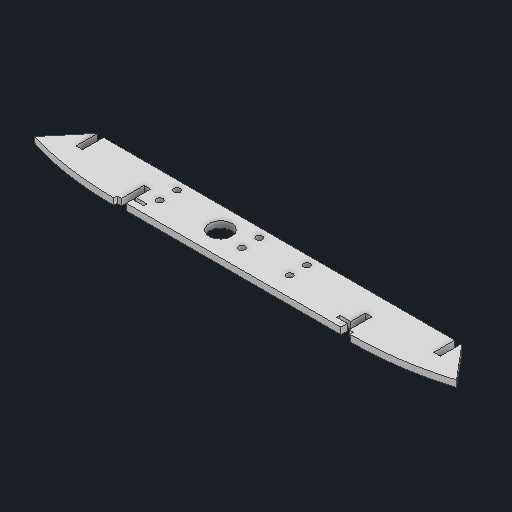
# Autodesk Inventor part: transom
Saved by Autodesk Inventor 2024 (Build 280153000, 153)
## iProperties
Created: 2022-03-21
Part Number: transom
Material: Generic
Document SubType Name: Modeling
Designer: kardo
Density: 1 g/cm^3
Appearance: Default
Mass: 10.6651 g
Surface Area: 88.9068 cm^2
Volume: 10.6651 cm^3
Author: kardo
Autodesk Inventor part; units mm, degrees
ref_plane "YZ Plane" through (0, 0, 0) normal (1, 0, 0) x (0, 1, 0)
ref_plane "XZ Plane" through (0, 0, 0) normal (0, 1, 0) x (-1, 0, 0)
ref_plane "XY Plane" through (0, 0, 0) normal (0, 0, 1) x (1, 0, 0)
derived "parameters_frame.ipt"
derived "stencil_frame.ipt"
sketch "sk_joint_locations" plane through (81.12, 0, 0) normal (1, 0, 0) x (0, 1, 0)
  line L0 (0, 0) -> (122.4, 9.6331) construction
  line L1 (36.465, 28.832) -> (112.2, 28.832) construction
  arc A0 (36.465, 28.832) -> (11.22, 28.376) centre (36.465, -670.197) ccw construction
  line L2 (-241.5001, 19.2432) -> (11.22, 28.376) construction
  line L3 (-345, 16.32) -> (-262.2001, 18.586) construction
  arc A1 (-262.2001, 18.586) -> (-241.5001, 19.2432) centre (-326.8578, 2381.2399) ccw construction
  line L4 (-122.4795, 3121.122) -> (270.8781, -1876.9598) construction
  line L5 (-230.0001, 3089.1136) -> (-230.0001, -1866.0023) construction
  line L6 (-114.9999, 3089.1136) -> (-114.9999, -1866.0023) construction
  line L7 (-345, 3089.1136) -> (-345, -1866.0023) construction
  line L8 (0, 3089.1136) -> (0, -1866.0023) construction
  line L9 (529.622, 47.2379) -> (-602.608, 2.7525) construction
  line L10 (-673.1615, -36.5999) -> (647.9226, 67.3717) construction
  line L11 (189.4528, 29.5173) -> (189.1111, 38.2146) construction
  line L12 (201.105, 36.5853) -> (201.7901, 27.8813) construction
  line L13 (0, 14.144) -> (121.9006, 15.9783) construction
  line L14 (-230.0001, 45.8224) -> (-230.0001, 19.6588) construction
  line L15 (-345, 37.3935) -> (-345, 16.32) construction
  line L16 (-114.9999, 50.9907) -> (-114.9999, 23.8147) construction
  line L17 (0, 52.89) -> (0, 27.9705) construction
  line L18 (119.1768, 50.5875) -> (119.7216, 43.6656) construction
  line L19 (120.2663, 36.7438) -> (119.7216, 43.6656) construction
  line L20 (120.2663, 36.7438) -> (120.8111, 29.822) construction
  line L21 (120.8111, 29.822) -> (121.3559, 22.9001) construction
  line L22 (121.3559, 22.9001) -> (121.9006, 15.9783) construction
  line L23 (0, 14.144) -> (0, 0) construction
  spline S0 degree 4 poles (-345, 37.3935) (-258.8686, 45.1235) (-172.5923, 49.7074) (-86.3167, 52.89) (0, 52.89) knots 0 0 0 0 0 1 1 1 1 1
  spline S1 degree 3 poles (0, 52.89) (92.8353, 52.89) (195.0311, 49.5089) (255, 36.448) knots 0 0 0 0 1 1 1 1
  spline S2 degree 2 poles (122.4, 9.6331) (190.08, 14.9596) (255, 36.448) knots 0 0 0 1 1 1
  line L24 (112.2, 37.536) -> (112.2, 28.832) construction
  line L25 (112.2, 35.848) -> (112.2, 30.52) construction
  point P0 (-122.4795, 3121.122)
  point P1 (270.8781, -1876.9598)
  point P2 (189.282, 33.8659)
  point P3 (201.4475, 32.2333)
  point P4 (134.9575, 11.3411)
  point P5 (-345, 26.8568)
  point P6 (-230.0001, 32.7406)
  point P7 (-114.9999, 37.4027)
  point P8 (0, 40.4303)
  point P9 (112.2, 33.184)
sketch "sk_rudder_mount" plane through (0, -345, 0) normal (0, 1, 0) x (-1, 0, 0)
  line L0 (54.6, -1866.0023) -> (54.6, 3089.1136) construction
  line L1 (0, 16.32) -> (54.6, 16.32) construction
  line L2 (43, 29.32) -> (43, 21.32) construction
  point P0 (0, 0)
  point P1 (0, 39.712)
sketch3d "sk_servo_rod"
sketch "sk_cowl_joint_locations" plane through (54.6, 0, 0) normal (1, 0, 0) x (0, 1, 0)
  line L0 (-345, 16.32) -> (-262.2001, 18.586) construction
  arc A0 (-262.2001, 18.586) -> (-241.5001, 19.2432) centre (-326.8578, 2381.2399) ccw construction
  line L1 (-241.5001, 19.2432) -> (11.22, 28.376) construction
  arc A1 (36.465, 28.832) -> (11.22, 28.376) centre (36.465, -670.197) ccw construction
  line L2 (36.465, 28.832) -> (112.2, 28.832) construction
  line L3 (94.8, 29.632) -> (36.465, 29.632) construction
  arc A2 (36.465, 29.632) -> (11.1911, 29.1755) centre (36.465, -670.197) ccw construction
  line L4 (11.1911, 29.1755) -> (-241.529, 20.0427) construction
  arc A3 (-262.222, 19.3857) -> (-241.529, 20.0427) centre (-326.8578, 2381.2399) ccw construction
  line L5 (-262.222, 19.3857) -> (-345, 17.1203) construction
  line L6 (-230.0001, 3089.1136) -> (-230.0001, -1866.0023) construction
  line L7 (-114.9999, 3089.1136) -> (-114.9999, -1866.0023) construction
  line L8 (-345, 3089.1136) -> (-345, -1866.0023) construction
  line L9 (0, 3089.1136) -> (0, -1866.0023) construction
  line L10 (-230.0001, 44.8681) -> (-230.0001, 20.4593) construction
  line L11 (-114.9999, 49.7658) -> (-114.9999, 24.6152) construction
  line L12 (-345, 17.1203) -> (-345, 17.1203)
  line L13 (-345, 17.1203) -> (-345, 36.7228) construction
  line L14 (-850.7464, 3011.9134) -> (325.2296, -1886.3794) construction
  line L15 (-344.7454, 36.7228) -> (-345, 39.712) construction
  line L16 (0, 51.4) -> (0, 28.7711) construction
  spline S0 degree 2 poles (-345, 39.712) (-172.656, 54.3934) (0, 54.4) knots 0 0 0 1 1 1
  spline S1 degree 3 poles (0, 54.4) (37.026, 54.4) (80.784, 47.9917) (112.2, 37.536) knots 1 1 1 1 2 2 2 2
  spline S2 degree 3 poles (111.2526, 34.6895) (106.0906, 36.4075) (96.4401, 39.2282) (84.5011, 42.0313) (75.2591, 43.9395) (68.9709, 45.1125) (60.9945, 46.449) (54.5373, 47.4124) (46.413, 48.4791) (39.8882, 49.2203) (31.7426, 50.0013) (25.2514, 50.5076) (17.2112, 50.9875) (9.2661, 51.3118) (3.0567, 51.4) (0, 51.4) knots 1 1 1 1 1.166667 1.291667 1.333333 1.416667 1.458333 1.541667 1.583333 1.666667 1.708333 1.791667 1.833333 1.916667 2 2 2 2
  spline S3 degree 3 poles (0, 51.4) (-19.1698, 51.3993) (-52.712, 51.1604) (-91.0357, 50.4121) (-119.7742, 49.6473) (-138.931, 49.0355) (-162.8744, 48.1436) (-182.0269, 47.3282) (-205.9648, 46.1816) (-225.113, 45.1626) (-249.0455, 43.7615) (-268.1894, 42.5387) (-292.1166, 40.883) (-316.041, 39.1) (-335.1777, 37.5379) (-344.7454, 36.7228) knots 0 0 0 0 0.166667 0.291667 0.333333 0.416667 0.458333 0.541666 0.583333 0.666666 0.708333 0.791666 0.833333 0.916666 1 1 1 1
  line L17 (-144.5331, 44.6212) -> (-139.5174, 23.7292) construction
  line L18 (-134.9371, 30.3529) -> (-140.7713, 28.9522) construction
  line L19 (-137.4449, 40.7989) -> (-143.2792, 39.3982) construction
  line L20 (-144.5331, 44.6212) -> (-138.6989, 46.0219) construction
  line L21 (-139.5174, 23.7292) -> (-133.6831, 25.1299) construction
  line L22 (-138.6989, 46.0219) -> (-138.9044, 52.0184) construction
  point P0 (0, 0)
  point P1 (-345, 26.9216)
  point P2 (-230.0001, 32.6637)
  point P3 (-114.9999, 37.1905)
  point P4 (0, 40.0855)
  point P5 (-850.7464, 3011.9134)
  point P6 (325.2296, -1886.3794)
  point P7 (-85.2629, 50.788)
  point P8 (0, 40.0855)
sketch "sk_strut_mount" plane through (0, -345, 0) normal (0, 1, 0) x (-1, 0, 0)
  line L0 (-6, -1866.0023) -> (-6, 3089.1136) construction
  line L1 (5, 21.32) -> (-17, 21.32) construction
  line L2 (5, 29.32) -> (-17, 29.32) construction
  line L3 (5, 21.32) -> (5, 29.32) construction
  line L4 (-17, 29.32) -> (-17, 21.32) construction
  point P0 (0, 0)
  point P1 (0, 39.712)
  point P2 (0, 16.32)
  point P3 (-6, 29.32)
  point P4 (-6, 21.32)
sketch "sk_transom_base" plane through (0, -345, 0) normal (0, 1, 0) x (-1, 0, 0)
  line L0 (-54.6, 39.712) -> (0, 39.712) construction
  spline S0 degree 2 poles (-54.6, 39.712) (-110.9753, 39.712) (-156, -0.1863) knots 0 0 0 1 1 1 construction
  line L1 (0, -1280.4843) -> (0, 2991.5273) construction
  line L2 (-54.6, -1280.4843) -> (-54.6, 2991.5273) construction
  line L3 (-81.12, -1280.4843) -> (-81.12, 2991.5273) construction
  line L4 (-1606.3078, 1829.616) -> (672.9966, -886.7531) construction
  line L5 (-97.4172, 32.6348) -> (-84.12, 16.7878)
  line L6 (-84.12, 16.7878) -> (-84.12, 26.8568)
  line L7 (-84.12, 26.8568) -> (-81.12, 26.8568)
  line L8 (-81.12, 26.8568) -> (-81.12, 17.12)
  line L9 (-81.12, 17.12) -> (0, 17.12)
  line L10 (0, 38.212) -> (0, 17.12)
  line L11 (-54.6, 38.912) -> (-54.6, 38.212)
  line L12 (-54.6, 38.212) -> (0, 38.212)
  spline S1 degree 5 poles (-54.6, 38.912) (-65.4969, 38.9115) (-76.3927, 37.9775) (-87.1849, 36.0074) (-108.6057, 29.8488) (-128.4524, 19.6871) (-138.0202, 13.5727) (-147.0181, 6.7042) (-155.4694, -0.785) knots 0 0 0 0 0 0 0.491099 0.491099 0.491099 1 1 1 1 1 1
  point P0 (0, 0)
  point P1 (-34.32, 16.32)
  dimension "d3" = 0.8
  dimension "d2" = 0.8
  dimension "d4" = 3
  dimension "d5" = 0.8
  dimension "d36" = 1.5
  constraints: 16 end point, 3 perpendicular, 2 collinear, 2 parallel, 2 point on line, 4 other
  measures "d2" distance between parallel lines of L4 L5
  measures "d4" distance of L6.end L7.end
  measures "d5" distance from line of L9 point (-34.32, 16.32)
  measures "d36" distance between parallel lines of L0 L12
extrude "thicken" add sketch "sk_transom_base" along normal blind 3
sketch "sk_cut_joint" plane through (0, -345, 0) normal (0, 1, 0) x (-1, 0, 0)
  line L0 (-54.6, 39.712) -> (0, 39.712) projected
  line L1 (-54.6, -1280.4843) -> (-54.6, 2991.5273) construction
  line L2 (-49.6, 39.712) -> (-49.6, 26.9216)
  line L3 (-49.6, 26.9216) -> (-52.6, 26.9216)
  line L4 (-52.6, 26.9216) -> (-52.6, 39.712)
  point P0 (0, 0)
  point P1 (-54.6, 26.9216)
  dimension "d25" = 3
  dimension "d26" = 5
  constraints: 6 end point, 3 parallel, 3 point on line
  measures "d25" distance between parallel lines of L2 L4
  measures "d26" distance between parallel lines of L2 L1
extrude "cut_joint" cut sketch "sk_cut_joint" along normal through all both and the other way through all
sketch "sk_cut_liner" plane through (0, -345, 0) normal (0, 1, 0) x (-1, 0, 0)
  line L0 (-54.6, 39.712) -> (0, 39.712) construction
  line L1 (-54.6, -1280.4843) -> (-54.6, 2991.5273) projected
  line L2 (-44.6, 39.712) -> (-44.6, 33.712)
  line L3 (-44.6, 33.712) -> (-49.6, 33.712)
  line L4 (-49.6, 33.712) -> (-49.6, 37.412)
  line L5 (-49.6, 37.412) -> (-54.6, 37.412)
  line L6 (-44.6, 35.212) -> (-49.6, 35.212)
  line L7 (-49.6, 39.712) -> (-49.6, 37.412)
  line L8 (-49.6, 39.712) -> (-54.6, 39.712)
  point P0 (0, 0)
  dimension "d29" = 5
  dimension "d30" = 5
  dimension "d32" = 2.3
  dimension "d33" = 1.5
  dimension "d37" = 6
  constraints: 14 end point, 6 parallel, 5 point on line
  measures "d29" distance between parallel lines of L1 L4
  measures "d30" distance between parallel lines of L4 L2
  measures "d32" distance between parallel lines of L0 L5
  measures "d33" distance between parallel lines of L3 L6
  measures "d37" distance between parallel lines of L0 L3
extrude "cut_liner" cut sketch "sk_cut_liner" along normal through all both and the other way through all
mirror "mirror" about plane through (0, 0, 0) normal (1, 0, 0)
hole "drill_rudder" at (-43, -345, 29.32) at (-43, -345, 21.32) direction (0, 1, 0) diameter 3 end through all
sketch "sk_servo_rod_drill" plane through (0, -345, 0) normal (0, 1, 0) x (-1, 0, 0)
  line L0 (15.1529, 28.2695) -> (17.1344, 27.1255) construction
  line L1 (0, -1280.4843) -> (0, 2991.5273) construction
  point P0 (0, 0)
  dimension "d38" = 2.288
  dimension "d53" = 60
  constraints: 2 end point, 1 coincident
  measures "d38" distance of L0.start L0.end
  measures "d53" angle of L1 L0
hole "drill_servo_rod" at (-17.1344, -345, 27.1255) direction (0, 1, 0) diameter 10.4 end through all
hole "drill_strut" at (-5, -345, 29.32) at (17, -345, 29.32) at (17, -345, 21.32) at (-5, -345, 21.32) direction (0, 1, 0) diameter 3 end through all
equation "\"d3\" = shell_thickness"
equation "\"d2\" = shell_thickness"
equation "\"d4\" = stringer_thickness"
equation "\"d5\" = shell_thickness"
equation "\"d36\" = cowl_shell_thickness"
equation "\"d7\" = bulkhead_thickness"
equation "\"d25\" = bulkhead_thickness"
equation "\"d26\" = cowl_liner_width"
equation "\"d29\" = cowl_liner_width"
equation "\"d30\" = cowl_sealing_width"
equation "\"d32\" = shell_thickness + cowl_liner_thickness"
equation "\"d33\" = cowl_liner_thickness"
equation "\"d37\" = cowl_sealing_thickness + cowl_shell_thickness + cowl_liner_thickness"
equation "\"d9\" = drill_rudder_mount_diam"
equation "\"d38\" = 0.22 * drill_servo_rod_diam"
equation "\"d39\" = drill_servo_rod_diam"
equation "\"d46\" = drill_struct_mount_diam"
equation "\"shell_thickness\" = 0.8"
equation "\"stringer_thickness\" = 3"
equation "\"cowl_shell_thickness\" = 1.5"
equation "\"bulkhead_thickness\" = 3"
equation "\"cowl_liner_width\" = 5"
equation "\"cowl_sealing_width\" = 5"
equation "\"cowl_liner_thickness\" = 1.5"
equation "\"cowl_sealing_thickness\" = 3"
equation "\"drill_rudder_mount_diam\" = 3"
equation "\"drill_servo_rod_diam\" = 10.4"
equation "\"drill_struct_mount_diam\" = 3"
body "Solid1"
